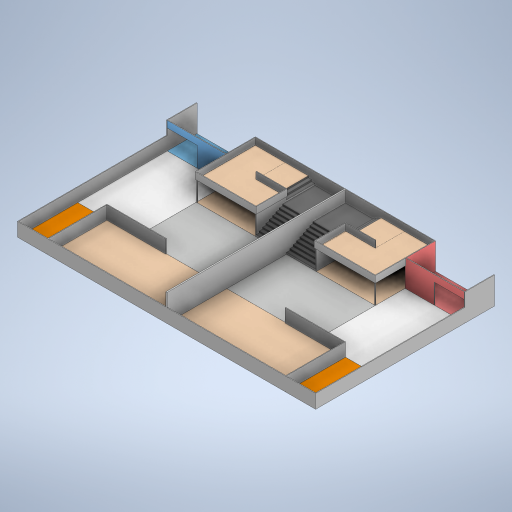
# Autodesk Inventor part: world
Saved by Autodesk Inventor 2024.1 (Build 281209000, 209)
## iProperties
Created: 2025-03-17
Part Number: world
Material: 一般
Document SubType Name: Modeling
Designer: hibik
Density: 1 g/cm^3
Appearance: 既定
Author: hibik
Autodesk Inventor part; units mm, degrees
ref_plane "YZ Plane" through (0, 0, 0) normal (1, 0, 0) x (0, 1, 0)
ref_plane "XZ Plane" through (0, 0, 0) normal (0, 1, 0) x (-1, 0, 0)
ref_plane "XY Plane" through (0, 0, 0) normal (0, 0, 1) x (1, 0, 0)
sketch "スケッチ1" plane through (0, 0, 0) normal (0, 1, 0) x (-1, 0, 0)
  line L0 (0, 0) -> (1800, 0)
  line L1 (1800, 0) -> (1800, 1800)
  line L2 (1800, 1800) -> (0, 1800) construction
  line L3 (0, 1800) -> (0, 0)
  line L4 (0, 1800) -> (1800, 1800) construction
  line L5 (1800, 1800) -> (1800, 3600)
  line L6 (1800, 3600) -> (0, 3600)
  line L7 (0, 3600) -> (0, 1800)
  line L8 (0, 3600) -> (900, 3600)
  line L9 (900, 3600) -> (900, 5400)
  line L10 (900, 5400) -> (0, 5400)
  line L11 (0, 5400) -> (0, 3600)
  line L12 (900, 5400) -> (4500, 5400)
  line L13 (4500, 5400) -> (4500, 3600)
  line L14 (4500, 3600) -> (900, 3600)
  line L15 (900, 3600) -> (900, 5400)
  line L16 (4500, 3600) -> (1800, 3600)
  line L17 (1800, 3600) -> (1800, 1800)
  line L18 (1800, 1800) -> (4500, 1800)
  line L19 (4500, 1800) -> (4500, 3600)
  line L20 (1800, 1800) -> (4500, 1800)
  line L21 (4500, 1800) -> (4500, 0)
  line L22 (4500, 0) -> (1800, 0)
  line L23 (1800, 0) -> (1800, 1800)
  line L24 (4500, 1800) -> (3600, 1800)
  line L25 (3600, 1800) -> (3600, 0)
  line L26 (3600, 0) -> (4500, 0)
  line L27 (4500, 0) -> (4500, 1800)
  line L28 (1800, 900) -> (0, 900)
  line L29 (1800, 899.9) -> (0, 899.9)
  line L30 (1799.9, 0) -> (1799.9, 899.9)
  line L31 (1800.1, 1800) -> (1800.1, 3600)
  line L32 (1800.1, 0) -> (1800.1, 1799.9)
  line L33 (1800.1, 1799.9) -> (3600, 1799.9)
  line L34 (1877.5864, 3600) -> (4500, 3600)
  line L35 (4500, 3600) -> (4500, 1864.0551)
  line L36 (3600, 1799.9) -> (4500, 1799.9)
  line L37 (4500, 3600.1) -> (0, 3600.1)
  line L38 (899.9, 3600.1) -> (899.9, 5400)
  point P0 (4500, 1800)
  point P1 (1800, 1799.9)
  point P2 (3600, 0)
  point P3 (900, 3600.1)
  dimension "d0" = 1800
  dimension "d1" = 1800
  dimension "d2" = 1800
  dimension "d3" = 1800
  dimension "d4" = 900
  dimension "d5" = 1800
  dimension "d6" = 3600
  dimension "d7" = 1800
  dimension "d8" = 900
  dimension "d9" = 1800
  dimension "d22" = 0.1
  dimension "d23" = 0.1
  dimension "d24" = 0.1
  dimension "d26" = 0.1
  dimension "d31" = 0.1
  dimension "d32" = 0.1
  dimension "d35" = 0.1
  dimension "d36" = 0.1
  constraints: 78 end point, 18 point on line, 15 parallel, 14 perpendicular, 7 horizontal, 2 midpoint
  measures "d0" distance of L2.end L1.end
  measures "d1" distance of L1.end L0.end
  measures "d2" distance of L6.end L5.end
  measures "d3" distance of L5.end L4.end
  measures "d4" distance of L10.end L9.end
  measures "d5" distance of L9.end L8.end
  measures "d6" distance of L13.end L14.end
  measures "d7" distance of L12.end L13.end
  measures "d8" distance of L26.end L25.end
  measures "d9" distance of L25.end L24.end
  measures "d22" distance between parallel lines of L29 L28
  measures "d23" distance between parallel lines of L30 L1
  measures "d24" distance between parallel lines of L5 L31
  measures "d26" distance between parallel lines of L18 L33
  measures "d31" distance between parallel lines of L32 L1
  measures "d32" distance between parallel lines of L24 L36
  measures "d35" distance between parallel lines of L8 L37
  measures "d36" distance between parallel lines of L9 L38
extrude "押し出し1" add sketch "スケッチ1" against normal blind 10 contours L3 L29 L30 L0
extrude "押し出し4" add sketch "スケッチ1" against normal blind 10 contours L32 L33 L25 L22 | L25 L36 L21 L22 | L9 L12 L13 L37
extrude "押し出し5" add sketch "スケッチ1" against normal blind 10 contours L3 L7 L6 L5 L1 L28
extrude "押し出し6" add sketch "スケッチ1" against normal blind 10 contours L31 L14 L19 L18
extrude "押し出し8" add sketch "スケッチ1" against normal blind 10 contours L11 L10 L38 L37
sketch "スケッチ4" plane through (0, 0, 0) normal (0, 1, 0) x (1, 0, 0)
  line L0 (-1800.1, -1799.9) -> (-1800.1, 0) projected
  line L1 (-1800.1, 0) -> (-4500, 0) projected
  line L2 (-4500, 0) -> (-4500, -1799.9) projected
  line L3 (-4500, -1799.9) -> (-1800.1, -1799.9) projected
  line L4 (-1800.1, -1799.9) -> (-1820.1, -1799.9)
  line L5 (-1820.1, -1799.9) -> (-1820.1, -1779.9)
  line L6 (-1820.1, -1779.9) -> (-1800.1, -1779.9)
  line L7 (-1800.1, -1779.9) -> (-1800.1, -1799.9)
  line L8 (-3600, -1799.9) -> (-3580, -1799.9)
  line L9 (-3580, -1799.9) -> (-3580, 0.1)
  line L10 (-3580, 0.1) -> (-3600, 0.1)
  line L11 (-3600, 0.1) -> (-3600, -1799.9)
  line L12 (-3600, -900) -> (-3580, -900)
  point P0 (0, 0)
  point P1 (-3600, 0)
  point P2 (-3580, 0)
  dimension "d41" = 20
  dimension "d42" = 20
  dimension "d43" = 20
  dimension "d44" = 1800
  dimension "d45" = 900
  dimension "d48" = 900
  constraints: 18 end point, 4 parallel, 3 perpendicular, 3 point on line, 2 horizontal
  measures "d41" distance of L5.end L6.end
  measures "d42" distance of L4.end L5.end
  measures "d43" distance of L10.end L9.end
  measures "d44" distance of L9.end L8.end
  measures "d45" distance between parallel lines of L2 L11
  measures "d48" distance between parallel lines of L1 L12
extrude "押し出し9" add sketch "スケッチ4" along normal blind 600 contours L3 L5 L6 L0 | L3 L11 L12 L9
sketch "スケッチ5" plane through (0, 600, 0) normal (0, 1, 0) x (1, 0, 0)
  line L0 (-3600, -900) -> (-3600, -1799.9) projected
  line L1 (-3580, -1799.9) -> (-1820.1, -1799.9) projected
  line L2 (-1800.1, -1800) -> (-4500, -1800) projected
  line L3 (-1800.1, -1779.9) -> (-1800.1, 0) projected
  line L4 (-3600, -1799.9) -> (-1800.1, -1799.9)
  line L5 (-1800.1, -1799.9) -> (-1800.1, 0)
  line L6 (-1800.1, 0) -> (-3600, 0)
  line L7 (-3600, 0) -> (-3600, -1799.9)
  line L8 (-3600, 0) -> (-2700, 0)
  line L9 (-2700, 0) -> (-2700, -900)
  line L10 (-2700, -900) -> (-3600, -900)
  line L11 (-3600, -900) -> (-3600, 0)
  point P0 (0, 0)
  dimension "d49" = 900
  dimension "d50" = 900
  constraints: 16 end point, 4 parallel, 2 horizontal, 2 perpendicular
  measures "d49" distance of L9.end L10.end
  measures "d50" distance of L8.end L9.end
extrude "押し出し10" add sketch "スケッチ5" against normal blind 5 contours L10 L9 L6 L3 L5 L4 L1 L0
sketch "スケッチ6" plane through (0, 0, 0) normal (0, 1, 0) x (1, 0, 0)
  line L0 (-1800.1, -1799.9) -> (-1800.1, 0) projected
  line L1 (0, 0) -> (-1799.9, 0) projected
  line L2 (-1799.9, 0) -> (-1779.9, 0)
  line L3 (-1779.9, 0) -> (-1779.9, -899.9)
  line L4 (-1779.9, -899.9) -> (-1799.9, -899.9)
  line L5 (-1799.9, -899.9) -> (-1799.9, 0)
  line L6 (-1799.9, -899.9) -> (0, -899.9) projected
  line L7 (0, -899.9) -> (0, 0) projected
  line L8 (0, 0) -> (-1799.9, 0) projected
  line L9 (-1799.9, 0) -> (-1799.9, -899.9) projected
  line L10 (-1799.9, -899.9) -> (-1799.9, 0) projected
  line L11 (0, -899.9) -> (-1779.9, -899.9)
  line L12 (-1779.9, -899.9) -> (-1779.9, -879.9)
  line L13 (-1779.9, -879.9) -> (0, -879.9)
  line L14 (0, -879.9) -> (0, -899.9)
  dimension "d53" = 20
  dimension "d54" = 20
  constraints: 16 end point, 4 parallel, 2 horizontal, 2 perpendicular, 1 point on line
  measures "d53" distance between parallel lines of L10 L3
  measures "d54" distance of L11.end L12.end
extrude "押し出し11" add sketch "スケッチ6" along normal blind 800 contours L3 L4 L5 L1 | L7 L6 L3 L13
sketch "スケッチ7" plane through (0, 600, 0) normal (0, 1, 0) x (1, 0, 0)
  line L0 (-1799.9, 0) -> (-1799.9, -899.9) projected
  line L1 (-3600, -1799.9) -> (-1800.1, -1799.9) projected
  line L2 (-1800.1, -1799.9) -> (-1800.1, 0) projected
  line L3 (-1800.1, 0) -> (-2700, 0) projected
  line L4 (-2700, 0) -> (-2700, -900) projected
  line L5 (-2700, -900) -> (-3600, -900) projected
  line L6 (-3600, -900) -> (-3600, -1799.9) projected
  line L7 (0, -899.9) -> (-1799.9, -899.9) projected
  line L8 (-1799.9, -899.9) -> (-1779.9, -899.9)
  line L9 (-1779.9, -899.9) -> (-1779.9, -1799.9)
  line L10 (-1779.9, -1799.9) -> (-1799.9, -1799.9)
  line L11 (-1799.9, -1799.9) -> (-1799.9, -899.9)
  line L12 (-1779.9, -879.9) -> (-1779.9, 0) projected
  line L13 (-1779.9, -1799.9) -> (-3620, -1799.9)
  line L14 (-3620, -1799.9) -> (-3620, -1819.9)
  line L15 (-3620, -1819.9) -> (-1779.9, -1819.9)
  line L16 (-1779.9, -1819.9) -> (-1779.9, -1799.9)
  line L17 (-3620, -1799.9) -> (-3600, -1799.9)
  line L18 (-3600, -1799.9) -> (-3600, -900)
  line L19 (-3600, -900) -> (-3620, -900)
  line L20 (-3620, -900) -> (-3620, -1799.9)
  line L21 (-2700, -900) -> (-3620, -900)
  line L22 (-3620, -900) -> (-3620, -880)
  line L23 (-3620, -880) -> (-2700, -880)
  line L24 (-2700, -880) -> (-2700, -900)
  line L25 (-1800.1, 0) -> (-4500, 0)
  line L26 (-4500, 0) -> (-4500, -20)
  line L27 (-4500, -20) -> (-1800.1, -20)
  line L28 (-1800.1, -20) -> (-1800.1, 0)
  line L29 (-4500, 0) -> (-4500, -1799.9) projected
  point P0 (0, 0)
  point P1 (-1800.1, -20)
  dimension "d57" = 20
  dimension "d58" = 20
  constraints: 40 end point, 10 parallel, 5 horizontal, 5 perpendicular, 2 collinear, 2 equal length, 2 point on line
  measures "d57" distance of L21.end L22.end
  measures "d58" distance between parallel lines of L20 L6
extrude "押し出し12" add sketch "スケッチ7" along normal blind 200 contours L13 L20 L19 L6 | L1 L13 L10 L16 L15 L14 | L19 L22 L23 L4 L5 | L27 L4 L3 L2 | L11 L7 L9 L10 | L27 L26 L25 L4
sketch "スケッチ8" plane through (0, 0, 0) normal (0, 1, 0) x (1, 0, 0)
  line L0 (-1800.1, -20) -> (-2700, -20) projected
  line L1 (-2700, -20) -> (-2700, -880) projected
  line L2 (-2700, -880) -> (-2700, -900) projected
  line L3 (-2700, -900) -> (-3600, -900) projected
  line L4 (-3600, -900) -> (-3600, -1799.9) projected
  line L5 (-3600, -1799.9) -> (-1800.1, -1799.9) projected
  line L6 (-1800.1, -1799.9) -> (-1800.1, -20) projected
  line L7 (-1820.1, -1799.9) -> (-1820.1, -1779.9) projected
  line L8 (-1820.1, -1779.9) -> (-1800.1, -1779.9) projected
  line L9 (-1800.1, -1779.9) -> (-1800.1, 0) projected
  line L10 (-1800.1, 0) -> (-4500, 0) projected
  line L11 (-4500, 0) -> (-4500, -1799.9) projected
  line L12 (-4500, -1799.9) -> (-3600, -1799.9) projected
  line L13 (-3600, -1799.9) -> (-3600, -900) projected
  line L14 (-3600, -900) -> (-3580, -900) projected
  line L15 (-3580, -900) -> (-3580, -1799.9) projected
  line L16 (-3580, -1799.9) -> (-1820.1, -1799.9) projected
  point P0 (0, 0)
extrude "押し出し13" add sketch "スケッチ8" along normal blind 450 contours L0 L1 L2 L3 L4 L12 L11 L10 L9
sketch "スケッチ9" plane through (-4500, -10, 0) normal (-1, 0, 0) x (0, 0, 1)
  line L0 (1800, 10) -> (3600, 10) projected
  line L1 (1800, 10) -> (1799.9, 60)
  line L2 (1799.9, 0) -> (1799.9, 460) projected
  line L3 (1699.9, 60) -> (1699.9, 110)
  line L4 (1699.9, 110) -> (1599.9, 110)
  line L5 (1599.9, 110) -> (1599.9, 160)
  line L6 (1599.9, 160) -> (1499.9, 160)
  line L7 (1499.9, 160) -> (1499.9, 210)
  line L8 (1499.9, 210) -> (1399.9, 210)
  line L9 (1399.9, 210) -> (1399.9, 260)
  line L10 (1399.9, 260) -> (1299.9, 260)
  line L11 (1299.9, 260) -> (1299.9, 310)
  line L12 (900, 460) -> (1799.9, 460) projected
  line L13 (1699.9, 60) -> (1799.9, 60)
  line L14 (1299.9, 310) -> (1199.9, 310)
  line L15 (1199.9, 310) -> (1199.9, 360)
  line L16 (1199.9, 360) -> (1099.9, 360)
  line L17 (1099.9, 360) -> (1099.9, 410)
  line L18 (1099.9, 410) -> (999.9, 410)
  line L19 (999.9, 410) -> (999.9, 460)
  line L20 (999.9, 460) -> (899.9, 460)
  point P0 (0, 10)
  dimension "d63" = 100
  dimension "d64" = 50
  dimension "d65" = 50
  constraints: 36 end point, 21 parallel, 6 perpendicular, 3 vertical, 2 horizontal, 1 point on line
  measures "d63" distance of L19.end L20.end
  measures "d64" distance of L18.end L19.end
  measures "d65" distance of L0.start L1.end
extrude "押し出し14" cut sketch "スケッチ9" against normal up to surface (900 mm away)
sketch "スケッチ10" plane through (0, 450, 0) normal (0, 1, 0) x (1, 0, 0)
  line L0 (-1800.1, -20) -> (-1800.1, 0) projected
  line L1 (-1800.1, 0) -> (-4500, 0) projected
  line L2 (-4500, 0) -> (-4500, -20) projected
  line L3 (-4500, -20) -> (-1800.1, -20) projected
  line L4 (-4500, -999.9) -> (-3600, -999.9) projected
  line L5 (-3600, -900) -> (-3600, -999.9) projected
  line L6 (-3580, -900) -> (-3600, -900) projected
  line L7 (-3580, -900) -> (-2700, -900) projected
  line L8 (-2700, -900) -> (-2700, -20) projected
  line L9 (-2700, -20) -> (-1800.1, -20) projected
  line L10 (-1800.1, -20) -> (-1800.1, 0) projected
  line L11 (-1800.1, 0) -> (-4500, 0) projected
  line L12 (-4500, 0) -> (-4500, -999.9) projected
  line L13 (-3600, -900) -> (-2700, -900)
  line L14 (-2700, -900) -> (-2700, -20)
  line L15 (-2700, -20) -> (-3600, -20)
  line L16 (-3600, -20) -> (-3600, -900)
  point P0 (0, 0)
  constraints: 8 end point, 2 parallel, 1 horizontal, 1 perpendicular
extrude "押し出し15" add sketch "スケッチ10" along normal up to surface (150 mm away) contours L3 L2 L1 L0 | L8 L7 L6 L16 L3
sketch "スケッチ11" plane through (-2700, 600, 880) normal (0, 0, -1) x (-1, 0, 0)
  line L0 (900, -150) -> (1800, -150) projected
  line L1 (1800, -150) -> (900, -150) projected
  line L2 (900, -150) -> (900, -100)
  line L3 (900, -100) -> (800, -100)
  line L4 (800, -100) -> (800, -50)
  line L5 (800, -50) -> (700, -50)
  line L6 (700, -50) -> (700, 0)
  line L7 (700, 0) -> (600, 0)
  line L8 (900, -200) -> (900, -150) projected
  line L9 (900, -250) -> (900, -200) projected
  line L10 (900, -300) -> (900, -250) projected
  line L11 (900, -350) -> (900, -300) projected
  line L12 (900, -400) -> (900, -350) projected
  line L13 (900, -450) -> (900, -400) projected
  line L14 (900, -500) -> (900, -450) projected
  line L15 (900, -550) -> (900, -500) projected
  line L16 (900, -550) -> (900, 0) projected
  line L17 (900, -150) -> (900, 0) projected
  line L18 (900, 0) -> (-899.9, 0) projected
  line L19 (0, 0) -> (900, 0) projected
  line L20 (0, 0) -> (900, 0) projected
  line L21 (900, 0) -> (-899.9, 0) projected
  point P0 (-2700, -600)
  point P1 (700, 0)
  dimension "d70" = 50
  dimension "d71" = 100
  constraints: 12 end point, 4 parallel, 3 perpendicular, 2 vertical, 1 horizontal
  measures "d70" distance of L1.end L2.end
  measures "d71" distance of L2.end L3.end
extrude "押し出し16" cut sketch "スケッチ11" along normal up to surface (860 mm away)
sketch "スケッチ12" plane through (0, 800, 0) normal (0, 1, 0) x (1, 0, 0)
  line L0 (0, 0) -> (-4500, 0)
  line L1 (-4500, 0) -> (-4500, -5400)
  line L2 (-4500, -5400) -> (0, -5400)
  line L3 (0, -5400) -> (0, 0)
  line L4 (-4480, 0) -> (-4480, -5400)
  line L5 (-20, 0) -> (-20, -5400)
  line L6 (-4500, -5380) -> (0, -5380)
  line L7 (-1800, -3600) -> (0, -3600) projected
  line L8 (-4500, -3600) -> (-1800.1, -3600) projected
  line L9 (-900, -5400) -> (-900, -3600.1) projected
  line L10 (-899.9, -5400) -> (-899.9, -3600.1) projected
  line L11 (-899.9, -3600.1) -> (-919.9, -3600.1)
  line L12 (-919.9, -3600.1) -> (-919.9, -5380)
  line L13 (-919.9, -5380) -> (-899.9, -5380)
  line L14 (-899.9, -5380) -> (-899.9, -3600.1)
  line L15 (-899.9, -3600.1) -> (-2699.9, -3600.1)
  line L16 (-2699.9, -3600.1) -> (-2699.9, -3620.1)
  line L17 (-2699.9, -3620.1) -> (-899.9, -3620.1)
  line L18 (-899.9, -3620.1) -> (-899.9, -3600.1)
  point P0 (-20, -5380)
  point P1 (-4480, -5380)
  point P2 (-919.9, -3620.1)
  point P3 (-900, -5380)
  dimension "d74" = 20
  dimension "d75" = 20
  dimension "d76" = 20
  dimension "d79" = 20
  dimension "d80" = 1800
  dimension "d81" = 20
  constraints: 30 end point, 6 parallel, 6 perpendicular, 6 point on line, 3 horizontal, 1 collinear
  measures "d74" distance between parallel lines of L2 L6
  measures "d75" distance between parallel lines of L3 L5
  measures "d76" distance between parallel lines of L1 L4
  measures "d79" distance of L13.end L12.end
  measures "d80" distance of L17.end L16.end
  measures "d81" distance of L16.end L15.end
extrude "押し出し17" add sketch "スケッチ12" against normal up to surface (800 mm away) contours L3 L7 L5 L0 | L3 L6 L5 L7 | L4 L8 L1 L0 | L3 L2 L5 L6 | L4 L6 L1 L8 | L5 L2 L10 L6 | L6 L9 L2 L4 | L4 L2 L1 L6 | L10 L2 L9 L6 | L12 L17 L9 L6 | L17 L16 L15 L12 | L12 L11 L9 L17
sketch "スケッチ13" plane through (0, 0, 0) normal (0, 1, 0) x (1, 0, 0)
  line L0 (-20, -879.9) -> (-920, -879.9)
  line L1 (-920, -879.9) -> (-920, -899.9)
  line L2 (-920, -899.9) -> (-20, -899.9)
  line L3 (-20, -899.9) -> (-20, -879.9)
  line L4 (-1779.9, -899.9) -> (-20, -899.9) projected
  point P0 (0, 0)
  dimension "d0" = 1800
  dimension "d1" = 1800
  dimension "d2" = 1800
  dimension "d3" = 1800
  dimension "d4" = 900
  dimension "d5" = 1800
  dimension "d6" = 3600
  dimension "d7" = 1800
  dimension "d8" = 900
  dimension "d9" = 1800
  dimension "d22" = 0.1
  dimension "d23" = 0.1
  dimension "d24" = 0.1
  dimension "d26" = 0.1
  dimension "d31" = 0.1
  dimension "d32" = 0.1
  dimension "d35" = 0.1
  dimension "d36" = 0.1
  dimension "d82" = 900
  constraints: 8 end point, 2 parallel, 1 collinear, 1 horizontal, 1 perpendicular
  measures "d82" distance of L2.end L1.end
extrude "押し出し18" cut sketch "スケッチ13" along normal blind 600
sketch "スケッチ14" plane through (0, -10, 0) normal (0, -1, 0) x (1, 0, 0)
  line L0 (-4500, 5400) -> (0, 5400) projected
  line L1 (-4500, 5400) -> (0, 5400)
  line L2 (0, 5400) -> (0, 0)
  line L3 (0, 0) -> (-4500, 0)
  line L4 (-4500, 0) -> (-4500, 5400)
  constraints: 8 end point, 2 parallel, 1 horizontal, 1 perpendicular
extrude "押し出し19" add sketch "スケッチ14" along normal mid plane 8
sketch "スケッチ15" plane through (0, 800, 0) normal (0, 1, 0) x (1, 0, 0)
  line L0 (-1779.9, -899.9) -> (-20, -899.9) projected
  line L1 (0, -5400) -> (0, 0) projected
  line L2 (0, -900) -> (-1800, -900) projected
  line L3 (0, -900) -> (-1779.9, -900)
  line L4 (-1779.9, -900) -> (-1779.9, -5400)
  line L5 (-1779.9, -5400) -> (0, -5400)
  line L6 (0, -5400) -> (0, -900)
  line L7 (-1779.9, -1819.9) -> (-1779.9, -899.9) projected
  line L8 (-4500, -5400) -> (0, -5400) projected
  line L9 (-4480, -5380) -> (-4480, -20) projected
  line L10 (0, -5400) -> (-4480, -5400)
  line L11 (-4480, -5400) -> (-4480, -3600.1)
  line L12 (-4480, -3600.1) -> (0, -3600.1)
  line L13 (0, -3600.1) -> (0, -5400)
  line L14 (-900, -3600.1) -> (-2699.9, -3600.1) projected
  point P0 (-9000, -5400)
  point P1 (-1779.9, -3600.1)
  constraints: 16 end point, 4 parallel, 3 collinear, 2 horizontal, 2 perpendicular, 1 point on line
extrude "押し出し20" cut sketch "スケッチ15" against normal blind 400
mirror "ミラー2" about plane through (-4500, 0, 3600) normal (-1, 0, 0)
equation "\"d58\" = d57"
